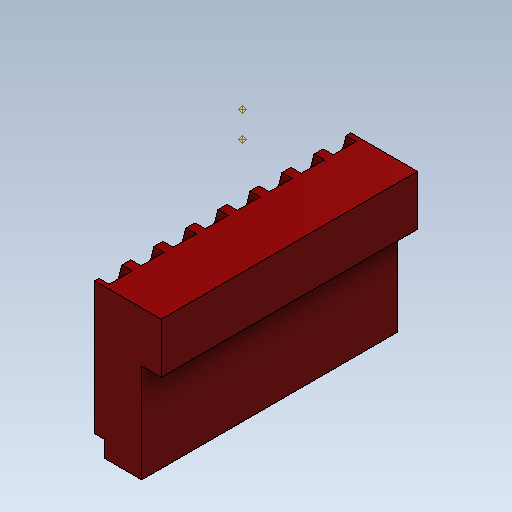
# Autodesk Inventor part: Connector, IDC, 8 Pin, SR
Saved by Autodesk Inventor 2020.1 (Build 241239000, 239)
## iProperties
GlobalPropertyList: <PropertyList/>
Created: 2005-11-07
Part Number: Connector, IDC, 8 Pin, SR
Document SubType Name: Modeling
Designer: Autodesk
Density: 1 g/cm^3
Mass: 3.34819 g
Surface Area: 22.2041 cm^2
Volume: 3.34819 cm^3
Categories: <MemberInstance><Categories><Category DisplayName="" Mnemonic="CABLEANDHARNESS" InternalName="e4a7e005-5e42-4d16-b293-125e7f0d0512"><Category DisplayName="" Mnemonic="CONNECTORS" InternalName="6f634eba-a678-4820-a31d-2c2d5ee6728e"><CategoryParameter DisplayName="" Mnemonic="REFDES" InternalName="c3740e8c-60ab-4d5d-8584-52b73222f2f0"/><Category DisplayName="" Mnemonic="DISCRETEWIRE" InternalName="9a3407de-09b2-4cdb-8c40-9708d5144a28"/></Category></Category></Categories><FamilyTemplate><FamilyTemplateParameters></FamilyTemplateParameters></FamilyTemplate><CategoryParameterMap><ParamToTemplateMap><ParamToTemplate CategoryParameter="//CategoryParameter[@InternalName='c3740e8c-60ab-4d5d-8584-52b73222f2f0']" ConstantValue=""/></ParamToTemplateMap></CategoryParameterMap></MemberInstance>
Material: Generic
Appearance: Red
Total Footprint: 0.000 kg
Author: Autodesk
Autodesk Inventor part; units mm, degrees
ref_plane "YZ Plane" through (0, 0, 0) normal (1, 0, 0) x (0, 1, 0)
ref_plane "XZ Plane" through (0, 0, 0) normal (0, 1, 0) x (-1, 0, 0)
ref_plane "XY Plane" through (0, 0, 0) normal (0, 0, 1) x (1, 0, 0)
sketch "Sketch1" plane through (0, 0, 0) normal (0, 0, 1) x (1, 0, 0)
  line L0 (-4.1275, 8.1915) -> (4.1275, 8.1915)
  line L1 (-4.1275, 8.1915) -> (-4.1275, -8.1915)
  line L2 (-2.8575, -10.2235) -> (1.7145, -10.2235)
  line L3 (-2.8575, -10.2235) -> (-2.8575, -8.1915)
  line L4 (-2.8575, -8.1915) -> (-4.1275, -8.1915)
  line L5 (4.1275, 8.1915) -> (4.1275, 1.9685)
  line L6 (1.7145, -10.2235) -> (1.7145, 1.9685)
  line L7 (4.1275, 1.9685) -> (1.7145, 1.9685)
  point P0 (0, 0)
  point P1 (0, 8.1915)
  point P2 (-4.1275, 0)
  dimension "d0" = 8.255
  dimension "d2" = 1.27
  dimension "d3" = 2.032
  dimension "d4" = 18.415
  dimension "d5" = 4.572
  dimension "d6" = 6.223
  constraints: 16 end point, 6 perpendicular, 2 midpoint, 1 horizontal, 1 horizontal alignment, 1 parallel, 1 vertical alignment
  measures "d0" distance of L0.start L0.end
  measures "d2" distance between parallel lines of L3 L1
  measures "d3" distance of L2.start L3.end
  measures "d4" distance between parallel lines of L2 L0
  measures "d5" distance of L2.start L2.end
  measures "d6" distance of L0.end L5.end
extrude "Extrusion1" add sketch "Sketch1" along normal blind 31.6992
sketch "Sketch2" plane through (-4.1275, -8.1915, 31.6992) normal (-1, 0, 0) x (0, 0, 1)
  line L0 (-31.6992, 16.383) -> (0, 16.383) projected
  line L1 (-31.6992, 0) -> (-31.6992, 16.383) projected
  line L2 (-31.6992, 0) -> (0, 0) projected
  line L3 (-31.115, 16.383) -> (-28.2702, 16.383)
  line L4 (-28.2702, 14.097) -> (-28.2702, 0)
  line L5 (-28.2702, 0) -> (-31.115, 0)
  line L6 (-31.115, 0) -> (-31.115, 14.097)
  line L7 (-30.5054, 14.605) -> (-30.5054, 14.097)
  line L8 (-31.115, 16.383) -> (-30.5054, 14.605)
  line L9 (-30.5054, 14.097) -> (-31.115, 14.097)
  line L10 (-28.8798, 14.605) -> (-28.8798, 14.097)
  line L11 (-28.2702, 16.383) -> (-28.8798, 14.605)
  line L12 (-28.8798, 14.097) -> (-28.2702, 14.097)
  line L13 (-27.1526, 16.383) -> (-24.3078, 16.383)
  line L14 (-24.3078, 14.097) -> (-24.3078, 0)
  line L15 (-24.3078, 0) -> (-27.1526, 0)
  line L16 (-27.1526, 0) -> (-27.1526, 14.097)
  line L17 (-26.543, 14.605) -> (-26.543, 14.097)
  line L18 (-27.1526, 16.383) -> (-26.543, 14.605)
  line L19 (-26.543, 14.097) -> (-27.1526, 14.097)
  line L20 (-24.3078, 16.383) -> (-24.9174, 14.605)
  line L21 (-24.9174, 14.605) -> (-24.9174, 14.097)
  line L22 (-24.9174, 14.097) -> (-24.3078, 14.097)
  line L23 (-23.1902, 16.383) -> (-20.3454, 16.383)
  line L24 (-20.3454, 14.097) -> (-20.3454, 0)
  line L25 (-20.3454, 0) -> (-23.1902, 0)
  line L26 (-23.1902, 0) -> (-23.1902, 14.097)
  line L27 (-22.5806, 14.605) -> (-22.5806, 14.097)
  line L28 (-23.1902, 16.383) -> (-22.5806, 14.605)
  line L29 (-22.5806, 14.097) -> (-23.1902, 14.097)
  line L30 (-20.3454, 16.383) -> (-20.955, 14.605)
  line L31 (-20.955, 14.605) -> (-20.955, 14.097)
  line L32 (-20.955, 14.097) -> (-20.3454, 14.097)
  line L33 (-19.2278, 16.383) -> (-16.383, 16.383)
  line L34 (-16.383, 14.097) -> (-16.383, 0)
  line L35 (-16.383, 0) -> (-19.2278, 0)
  line L36 (-19.2278, 0) -> (-19.2278, 14.097)
  line L37 (-18.6182, 14.605) -> (-18.6182, 14.097)
  line L38 (-19.2278, 16.383) -> (-18.6182, 14.605)
  line L39 (-18.6182, 14.097) -> (-19.2278, 14.097)
  line L40 (-16.383, 16.383) -> (-16.9926, 14.605)
  line L41 (-16.9926, 14.605) -> (-16.9926, 14.097)
  line L42 (-16.9926, 14.097) -> (-16.383, 14.097)
  line L43 (-15.2654, 16.383) -> (-12.4206, 16.383)
  line L44 (-12.4206, 14.097) -> (-12.4206, 0)
  line L45 (-12.4206, 0) -> (-15.2654, 0)
  line L46 (-15.2654, 0) -> (-15.2654, 14.097)
  line L47 (-14.6558, 14.605) -> (-14.6558, 14.097)
  line L48 (-15.2654, 16.383) -> (-14.6558, 14.605)
  line L49 (-14.6558, 14.097) -> (-15.2654, 14.097)
  line L50 (-12.4206, 16.383) -> (-13.0302, 14.605)
  line L51 (-13.0302, 14.605) -> (-13.0302, 14.097)
  line L52 (-13.0302, 14.097) -> (-12.4206, 14.097)
  line L53 (-11.303, 16.383) -> (-8.4582, 16.383)
  line L54 (-8.4582, 14.097) -> (-8.4582, 0)
  line L55 (-8.4582, 0) -> (-11.303, 0)
  line L56 (-11.303, 0) -> (-11.303, 14.097)
  line L57 (-10.6934, 14.605) -> (-10.6934, 14.097)
  line L58 (-11.303, 16.383) -> (-10.6934, 14.605)
  line L59 (-10.6934, 14.097) -> (-11.303, 14.097)
  line L60 (-8.4582, 16.383) -> (-9.0678, 14.605)
  line L61 (-9.0678, 14.605) -> (-9.0678, 14.097)
  line L62 (-9.0678, 14.097) -> (-8.4582, 14.097)
  line L63 (-7.3406, 16.383) -> (-4.4958, 16.383)
  line L64 (-4.4958, 14.097) -> (-4.4958, 0)
  line L65 (-4.4958, 0) -> (-7.3406, 0)
  line L66 (-7.3406, 0) -> (-7.3406, 14.097)
  line L67 (-6.731, 14.605) -> (-6.731, 14.097)
  line L68 (-7.3406, 16.383) -> (-6.731, 14.605)
  line L69 (-6.731, 14.097) -> (-7.3406, 14.097)
  line L70 (-4.4958, 16.383) -> (-5.1054, 14.605)
  line L71 (-5.1054, 14.605) -> (-5.1054, 14.097)
  line L72 (-5.1054, 14.097) -> (-4.4958, 14.097)
  line L73 (-3.3782, 16.383) -> (-0.5334, 16.383)
  line L74 (-0.5334, 14.097) -> (-0.5334, 0)
  line L75 (-0.5334, 0) -> (-3.3782, 0)
  line L76 (-3.3782, 0) -> (-3.3782, 14.097)
  line L77 (-2.7686, 14.605) -> (-2.7686, 14.097)
  line L78 (-3.3782, 16.383) -> (-2.7686, 14.605)
  line L79 (-2.7686, 14.097) -> (-3.3782, 14.097)
  line L80 (-0.5334, 16.383) -> (-1.143, 14.605)
  line L81 (-1.143, 14.605) -> (-1.143, 14.097)
  line L82 (-1.143, 14.097) -> (-0.5334, 14.097)
  dimension "d9" = 0.5842
  dimension "d10" = 2.8448
  dimension "d11" = 0.6096
  dimension "d12" = 0.508
  dimension "d13" = 2.286
  dimension "d14" = 2.286
  dimension "d15" = 0.508
  dimension "d18" = 3.9624
  constraints: 160 end point, 3 parallel, 2 horizontal, 2 perpendicular, 2 point on line, 140 other
  measures "d9" distance between parallel lines of L6 L1
  measures "d10" distance between parallel lines of L4 L6
  measures "d11" distance of L7.end L6.end
  measures "d12" distance of L7.start L7.end
  measures "d13" distance between parallel lines of L0 L9
  measures "d14" distance between parallel lines of L3 L12
  measures "d15" distance of L11.end L10.end
  measures "d18" distance of L5.end L16.start
extrude "Extrusion2" cut sketch "Sketch2" against normal blind 1.27 contours L0 L11 L10 L12 L4 L2 L6 L9 L7 L8 | L0 L20 L21 L22 L14 L2 L16 L19 L17 L18 | L0 L30 L31 L32 L24 L2 L26 L29 L27 L28 | L0 L40 L41 L42 L34 L2 L36 L39 L37 L38 | L0 L50 L51 L52 L44 L2 L46 L49 L47 L48 | L0 L60 L61 L62 L54 L2 L56 L59 L57 L58 | L0 L70 L71 L72 L64 L2 L66 L69 L67 L68 | L0 L80 L81 L82 L74 L2 L76 L79 L77 L78
body "Solid1"
